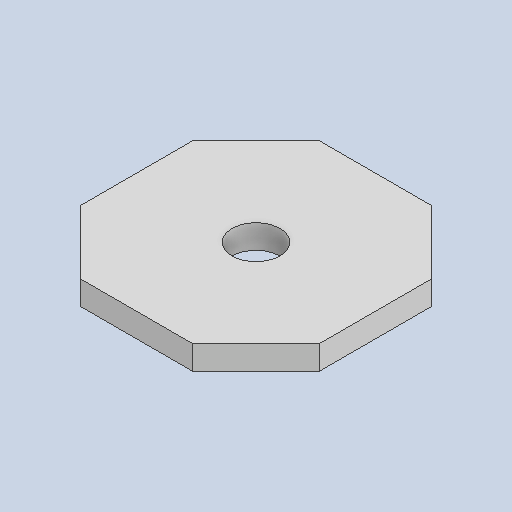
# Autodesk Inventor part: chamber_base
Saved by Autodesk Inventor 2025.4 (Build 294407000, 407)
## iProperties
Created: 2026-05-14
Part Number: chamber_base
Material: Generic
Document SubType Name: Modeling
Designer: zboichykb
Density: 1 g/cm^3
Appearance: Default
Author: zboichykb
Autodesk Inventor part; units mm, degrees
ref_plane "YZ Plane" through (0, 0, 0) normal (1, 0, 0) x (0, 1, 0)
ref_plane "XZ Plane" through (0, 0, 0) normal (0, 1, 0) x (-1, 0, 0)
ref_plane "XY Plane" through (0, 0, 0) normal (0, 0, 1) x (1, 0, 0)
sketch "Sketch1" plane through (0, 0, 0) normal (0, 1, 0) x (-1, 0, 0)
  line L0 (0, 0) -> (254, 0)
  line L1 (254, 0) -> (254, -119.38)
  line L2 (254, -119.38) -> (0, -119.38)
  line L3 (0, -119.38) -> (0, 0)
  line L4 (186.69, 67.31) -> (67.31, 67.31)
  line L5 (67.31, 67.31) -> (67.31, -186.69)
  line L6 (67.31, -186.69) -> (186.69, -186.69)
  line L7 (186.69, -186.69) -> (186.69, 67.31)
  line L8 (186.69, 67.31) -> (254, 0)
  line L9 (67.31, 67.31) -> (0, 0)
  line L10 (186.69, -186.69) -> (254, -119.38)
  line L11 (0, -119.38) -> (67.31, -186.69)
  line L12 (62.2907, -7.1202) -> (161.0967, -7.1202)
  line L13 (164.2717, -10.2952) -> (164.2717, -109.1012)
  line L14 (161.0967, -112.2762) -> (62.2907, -112.2762)
  line L15 (59.1157, -109.1012) -> (59.1157, -10.2952)
  arc A0 (62.2907, -7.1202) -> (59.1157, -10.2952) centre (62.2907, -10.2952) ccw
  arc A1 (164.2717, -10.2952) -> (161.0967, -7.1202) centre (161.0967, -10.2952) ccw
  arc A2 (161.0967, -112.2762) -> (164.2717, -109.1012) centre (161.0967, -109.1012) ccw
  arc A3 (59.1157, -109.1012) -> (62.2907, -112.2762) centre (62.2907, -109.1012) ccw
  point P0 (164.2717, -112.2762)
  point P1 (164.2717, -7.1202)
  point P2 (59.1157, -112.2762)
  dimension "d0" = 254
  dimension "d1" = 119.38
  dimension "d2" = 119.38
  dimension "d3" = 254
  dimension "d8" = 95.1907
  dimension "d14" = 105.156
  dimension "d15" = 105.156
  dimension "d22" = 3.175
  constraints: 32 end point, 8 point on circle, 8 tangent, 7 parallel, 6 point on line, 4 centre point, 3 equal radius, 3 horizontal, 3 perpendicular, 1 coincident
  measures "d0" distance of L1.end L2.end
  measures "d1" distance of L0.end L1.end
  measures "d2" distance of L6.end L5.end
  measures "d3" distance of L5.end L4.end
  measures "d8" distance of L0.end L4.start
  measures "d14" distance of point (164.272, -112.276) point (59.116, -112.276)
  measures "d15" distance of point (164.272, -7.12) point (164.272, -112.276)
  measures "d22" radius of A0
extrude "Extrusion1" add sketch "Sketch1" along normal blind 25.4
sketch "Sketch4" plane through (0, 25.4, 0) normal (0, 1, 0) x (1, 0, 0)
  circle A0 centre (-127, 59.69) radius 25.4
  line L0 (-254, 59.69) -> (-127, 59.69)
  line L1 (-127, 59.69) -> (-127, 186.69)
  line L2 (-254, 119.38) -> (-254, 0) projected
  line L3 (-67.31, 186.69) -> (-186.69, 186.69) projected
  point P0 (0, 0)
  dimension "d50" = 50.8
  dimension "d58" = 127
  dimension "d59" = 127
  constraints: 7 coincident, 4 end point, 3 midpoint, 1 centre point, 1 horizontal, 1 vertical
  measures "d50" diameter of A0
  measures "d58" distance of L0.start L0.end
  measures "d59" distance of L1.end L1.start
extrude "Extrusion3" cut sketch "Sketch4" against normal blind 25.4
equation "\"d0\" = rectangle_L"
equation "\"d1\" = rectangle_01_w"
equation "\"d2\" = rectangle_01_w"
equation "\"d3\" = rectangle_L"
equation "\"d8\" = d9"
equation "\"d14\" = window_L"
equation "\"d15\" = window_L"
equation "\"rectangle_L\" = 254"
equation "\"rectangle_01_w\" = 119.38"
equation "\"d9\" = 95.19071"
equation "\"window_L\" = 105.156"
equation "\"test\" = 74.422"
equation "\"electrode_diam\" = 50.8"
equation "\"test_points\" = 127"
body "Solid1"
